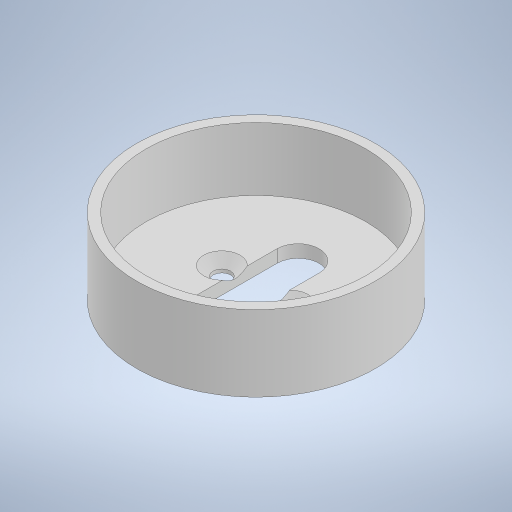
# Autodesk Inventor part: кроватка
Saved by Autodesk Inventor 2023.1 (Build 271208000, 208)
## iProperties
Created: 2025-03-30
Part Number: кроватка
Material: Типовые
Document SubType Name: Modeling
Designer: DELL
Density: 1 g/cm^3
Appearance: По умолчанию
Author: DELL
Autodesk Inventor part; units mm, degrees
ref_plane "YZ Plane" through (0, 0, 0) normal (1, 0, 0) x (0, 1, 0)
ref_plane "XZ Plane" through (0, 0, 0) normal (0, 1, 0) x (-1, 0, 0)
ref_plane "XY Plane" through (0, 0, 0) normal (0, 0, 1) x (1, 0, 0)
sketch "Эскиз1" plane through (0, 0, 0) normal (0, 0, 1) x (1, 0, 0)
  line L0 (0, 0) -> (-28.3405, 0)
  line L1 (-28.3405, 0) -> (-28.3405, 3)
  line L2 (-28.3405, 3) -> (0, 3)
  line L3 (0, 3) -> (0, 0)
  line L4 (-28.3405, 0) -> (-26.0995, 0)
  line L5 (-26.0995, 0) -> (-26.0995, 18)
  line L6 (-26.0995, 18) -> (-28.3405, 18)
  line L7 (-28.3405, 18) -> (-28.3405, 0)
  line L8 (0, -3.6) -> (0, 21.6) projected
  point P0 (-26.0995, 3)
  dimension "d0" = 28.3405
  dimension "d1" = 3
  dimension "d2" = 2.241
  dimension "d3" = 18
  constraints: 16 end point, 4 parallel, 2 horizontal, 2 perpendicular
  measures "d0" distance of L1.end L2.end
  measures "d1" distance of L0.end L1.end
  measures "d2" distance of L6.end L5.end
  measures "d3" distance of L5.end L4.end
revolve "Вращение1" add sketch "Эскиз1" angle 360 about axis through (0, -10, 0) along (0, 1, 0)
sketch "Эскиз2" plane through (0, 3, 0) normal (0, 1, 0) x (1, 0, 0)
  line L0 (0, 10) -> (0, -10) construction
  line L1 (-5, 10) -> (-5, -10)
  line L2 (5, -10) -> (5, 10)
  arc A0 (5, 10) -> (-5, 10) centre (0, 10) ccw
  arc A1 (-5, -10) -> (5, -10) centre (0, -10) ccw
  circle A2 centre (8.1, 0) radius 2.1
  circle A3 centre (-8.1, 0) radius 2.1
  point P0 (0, 0)
  dimension "d5" = 10
  dimension "d6" = 10
  dimension "d7" = 4.2
  dimension "d8" = 3.1
  constraints: 8 end point, 4 centre point, 4 point on circle, 4 tangent, 1 midpoint, 1 parallel, 1 symmetric about line, 1 vertical, 1 other
  measures "d5" distance of point (0, 0) L0.end
  measures "d6" diameter of A1
  measures "d7" diameter of A2
  measures "d8" distance from line of L2 A2.centre
extrude "Выдавливание1" cut sketch "Эскиз2" against normal blind 10
chamfer "Фаска1" distance 2.2 angle 45 1 edges at (-10.2, 3, 0)
chamfer "Фаска2" distance 2.2 angle 45 1 edges at (6, 3, 0)
